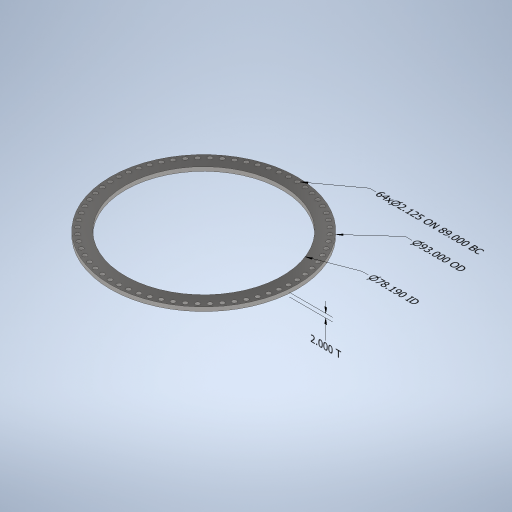
# Autodesk Inventor part: AWWA C207-18 Class B Ring and Blind Flange
Saved by Autodesk Inventor 2023 (Build 270158000, 158)
## iProperties
RuleStatus: InUse
Created: 2023-06-05
Part Number: AWWA C207-18 Class B Ring and Blind Flange
Material: Generic
Document SubType Name: Modeling
Designer: Admin
Density: 1 g/cm^3
Appearance: Steel - Polished
Author: Admin
Autodesk Inventor part; units mm, degrees
ref_plane "YZ Plane" through (0, 0, 0) normal (1, 0, 0) x (0, 1, 0)
ref_plane "XZ Plane" through (0, 0, 0) normal (0, 1, 0) x (-1, 0, 0)
ref_plane "XY Plane" through (0, 0, 0) normal (0, 0, 1) x (1, 0, 0)
sketch "Flange Sketch" plane through (0, 0, 0) normal (0, 1, 0) x (-1, 0, 0)
  circle A0 centre (0, 0) radius 1181.1
  circle A1 centre (0, 0) radius 993.013
  circle A2 centre (0, 0) radius 1130.3 construction
  line L0 (0, 0) -> (-55.4612, -1128.9385) construction
  line L1 (0, 0) -> (0, -1130.3) construction
  dimension "outerDiam" = 2362.2
  dimension "innerDiam" = 1986.026
  dimension "boltCircle" = 2260.6
  dimension "boltOffsetAngle" = 2.812
  constraints: 4 end point, 3 centre point, 3 coincident, 2 point on circle, 1 vertical
  measures "outerDiam" diameter of A0
  measures "innerDiam" diameter of A1
  measures "boltCircle" diameter of A2
  measures "boltOffsetAngle" angle of L0 L1
extrude "Flange Extrusion" add sketch "Flange Sketch" along normal blind 50.8
hole "Bolt Hole" at (55.4612, 0, -1128.9385) direction (0, 1, 0) diameter 53.975 depth 50.8
pattern_circular "Bolt Hole Pattern" count 64 over 360 about axis through (0, -10, 0) along (0, 1, 0) of "Bolt Hole"
equation "\"nominalSize\" = 1981.2"
body "Solid1"
